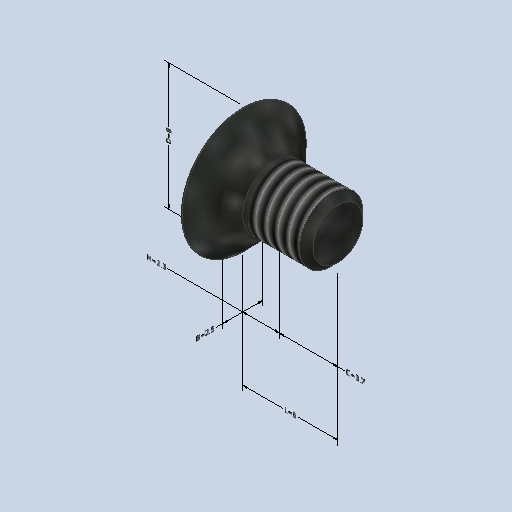
# Autodesk Inventor part: FBB4-6
Saved by Autodesk Inventor 2023 (Build 270158000, 158)
## iProperties
Category: PARTsolutions
Company: TOHATSU
Created: 2023-07-22
Part Number: FBB4-6
Material: Steel
Catalog Web Link: www.cadenas.de
Description: FBB SFBB-Pan head hexagon socket screw
Vendor: TOHATSU
Document SubType Name: Modeling
Designer: psAdmin
Manufacturer: TOHATSU
Mass: 0.79702 g
Surface Area: 1.69878 cm^2
Volume: 0.101531 cm^3
Density: 7.85 g/cm^3
Appearance: Plate
PSOL_IDENT_0: {$CADENAS_DATA/23d-libs/tohatsu/spring_screw_washer/screws_bolts_nuts/screws_bolts/fbb.prj},161 {VTY
PSOL_IDENT_1: P=3D},{NB=FBB4-6},{LINA=FBB4-6},{NN=FBB SFBB},{DATE=19.07.2023 02:54:23},{GEOMDATE=08.12.2022 08:35:
PSOL_IDENT_2: 03},{VERSION=},{LINEID=20},{WBVAR=TYPE,L},{WBNUMERIC=L}  {NB=FBB4-6},{LINA=FBB4-6},{KT=DUMMY},{PN=FB
PSOL_IDENT_3: B4-6},{ROHS=YES},{TYPE=FBB},{MA=SCM435},{QU=7810},{COL=0.30,0.35,0.36,0.00},{M=4},{L=6},{DIML=6,8,10
PSOL_IDENT_4: ,12,16,20,25},{P=0.70},{MXP=M4X0.7},{D=8.0},{H=2.3},{B=2.5},{C=3.7},{URL=https://www.tohatsu.com.tw}
PSOL_IDENT_5: ,{WED=網站}
NB: FBB4-6
NN: FBB SFBB
NT: Pan head hexagon socket screw
NBSYN: $PN.
LINA: FBB4-6
CATALOG: TOHATSU
PN: FBB4-6
ROHS: YES
TYPE: FBB
MA: SCM435
M: 4
L: 6
WED: 網站
SUPPLIER: TOHATSU
ARTICLENO: FBB4-6
BOMINFO: FBB4-6
CREATOR: CADENAS GmbH
Title: FBB4-6
Author: Cadenas PARTsolutions
Comments: Pan head hexagon socket screw
Autodesk Inventor part; units mm, degrees
ref_plane "YZ Plane" through (0, 0, 0) normal (1, 0, 0) x (0, 1, 0)
ref_plane "XZ Plane" through (0, 0, 0) normal (0, 1, 0) x (-1, 0, 0)
ref_plane "XY Plane" through (0, 0, 0) normal (0, 0, 1) x (1, 0, 0)
sketch "__1" plane through (0, 0, 0) normal (0, 0, 1) x (1, 0, 0)
  line L0 (56, 0) -> (-56, 0)
  line L1 (0, 0) -> (0, 4)
  line L2 (0, 4) -> (2, 2)
  line L3 (2, 2) -> (5.5705, 2)
  line L4 (5.5705, 2) -> (6, 1.5705)
  line L5 (6, 1.5705) -> (6, 0)
  line L6 (6, 0) -> (0, 0)
  constraints: 14 end point
revolve "Revolution1" add sketch "__1" angle 360 about axis through (56, 0, 0) along (1, 0, 0)
thread "Thread1" size "M4x0.7" class "6g" standard "ISO Metric profile" length 3.2705
sketch "__2" plane through (0, 0, 0) normal (1, 0, 0) x (0, 0, -1)
  line L0 (-1.25, -0.7217) -> (0, -1.4434)
  line L1 (0, -1.4434) -> (1.25, -0.7217)
  line L2 (1.25, -0.7217) -> (1.25, 0.7217)
  line L3 (1.25, 0.7217) -> (0, 1.4434)
  line L4 (0, 1.4434) -> (-1.25, 0.7217)
  line L5 (-1.25, 0.7217) -> (-1.25, -0.7217)
  constraints: 12 end point
extrude "Extrusion1" cut sketch "__2" along normal blind 1.15
fillet "Fillet1" radius 0.05 1 edges at (0, -4, 0)
body "Solid1"
